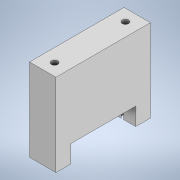
# Autodesk Inventor part: LowerJawSupport
Saved by Autodesk Inventor 2022 (Build 260153000, 153)
## iProperties
Created: 2021-11-02
Part Number: LowerJawSupport
Material: Genérico
Document SubType Name: Modeling
Designer: JK
Density: 1 g/cm^3
Appearance: Valor por defecto
Author: JK
Autodesk Inventor part; units mm, degrees
ref_plane "YZ Plane" through (0, 0, 0) normal (1, 0, 0) x (0, 1, 0)
ref_plane "XZ Plane" through (0, 0, 0) normal (0, 1, 0) x (-1, 0, 0)
ref_plane "XY Plane" through (0, 0, 0) normal (0, 0, 1) x (1, 0, 0)
sketch "Boceto1" plane through (0, 0, 0) normal (0, 1, 0) x (-1, 0, 0)
  line L0 (-11.1918, 40) -> (11.1918, 40)
  line L1 (11.1918, 40) -> (11.1918, -40)
  line L2 (11.1918, -40) -> (-11.1918, -40)
  line L3 (-11.1918, -40) -> (-11.1918, 40)
  line L4 (-11.1918, 40) -> (11.1918, -40) construction
  line L5 (11.1918, 40) -> (-11.1918, -40) construction
  circle A0 centre (0, 30) radius 2.7
  circle A1 centre (0, -30) radius 2.7
  point P0 (0, 0)
  dimension "d0" = 5.4
  dimension "d1" = 80
  dimension "d2" = 10
  dimension "d3" = 10
  constraints: 12 end point, 2 centre point, 2 midpoint, 2 parallel, 1 equal radius, 1 horizontal, 1 perpendicular
  measures "d0" diameter of A0
  measures "d1" distance of L0.end L1.end
  measures "d2" distance from line of L0 A0.centre
  measures "d3" distance from line of L2 A1.centre
extrude "Extrusión1" add sketch "Boceto1" along normal blind 70
sketch "Boceto2" plane through (-11.1918, 0, -40) normal (-1, 0, 0) x (0, 0, 1)
  line L0 (67.5, -15) -> (12.5, -15)
  line L1 (12.5, -15) -> (12.5, 15)
  line L2 (12.5, 15) -> (67.5, 15)
  line L3 (67.5, 15) -> (67.5, -15)
  line L4 (67.5, -15) -> (12.5, 15) construction
  line L5 (12.5, -15) -> (67.5, 15) construction
  point P0 (40, 0)
  dimension "d6" = 55
  dimension "d7" = 30
  constraints: 12 end point, 2 midpoint, 2 parallel, 1 horizontal, 1 perpendicular
  measures "d6" distance between parallel lines of L3 L1
  measures "d7" distance of L0.end L1.end
extrude "Extrusión2" cut sketch "Boceto2" against normal through all
